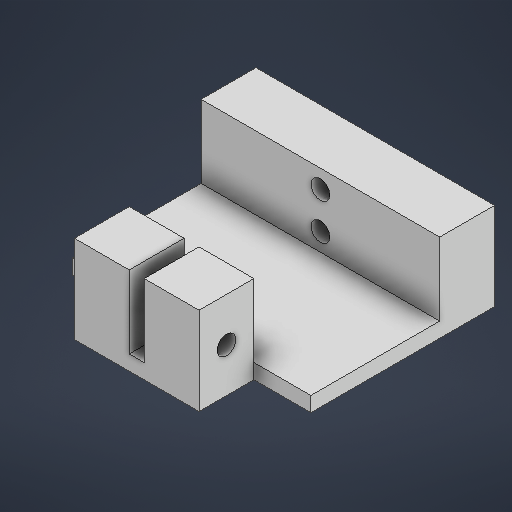
# Autodesk Inventor part: Slit holder
Saved by Autodesk Inventor 2027 (Build 310192060, 192F)
## iProperties
Created: 2026-07-27
Part Number: Slit holder
Material: Generic
Document SubType Name: Modeling
Designer: blaze
Density: 1 g/cm^3
Appearance: Default
Author: blaze
Autodesk Inventor part; units mm, degrees
ref_plane "YZ Plane" through (0, 0, 0) normal (1, 0, 0) x (0, 1, 0)
ref_plane "XZ Plane" through (0, 0, 0) normal (0, 1, 0) x (-1, 0, 0)
ref_plane "XY Plane" through (0, 0, 0) normal (0, 0, 1) x (1, 0, 0)
sketch "Sketch1" plane through (0, 0, 0) normal (0, 0, 1) x (1, 0, 0)
  line L0 (0, 0) -> (50.8, 0)
  line L1 (50.8, 0) -> (50.8, 18.669)
  line L2 (50.8, 18.669) -> (0, 18.669)
  line L3 (0, 18.669) -> (0, 0)
  dimension "d0" = 50.8
  dimension "d1" = 18.669
  constraints: 8 end point, 2 parallel, 1 horizontal, 1 perpendicular
  measures "d0" distance of L2.end L1.end
  measures "d1" distance of L1.end L0.end
extrude "Extrusion1" add sketch "Sketch1" against normal blind 50.8
sketch "Sketch2" plane through (0, 0, 0) normal (0, 0, 1) x (1, 0, 0)
  line L0 (50.8, 0) -> (0, 0) projected
  line L1 (25.4, 0) -> (25.4, 3.175)
  line L2 (25.4, 3.175) -> (26.9875, 3.175)
  line L3 (25.4, 3.175) -> (23.8125, 3.175)
  line L4 (23.8125, 3.175) -> (23.8125, 18.669)
  line L5 (0, 18.669) -> (50.8, 18.669) projected
  line L6 (26.9875, 3.175) -> (26.9875, 18.669)
  line L7 (23.8125, 18.669) -> (12.1285, 18.669)
  line L8 (12.1285, 18.669) -> (12.1285, 0)
  line L9 (12.1285, 0) -> (25.4, 0)
  line L10 (26.9875, 18.669) -> (38.6715, 18.669)
  line L11 (38.6715, 18.669) -> (38.6715, 0)
  line L12 (38.6715, 0) -> (25.4, 0)
  line L13 (0, 0) -> (0, 18.669) projected
  line L14 (0, 18.669) -> (0, 0)
  line L15 (50.8, 18.669) -> (50.8, 0) projected
  line L16 (50.8, 18.669) -> (50.8, 0)
  dimension "d4" = 3.175
  dimension "d5" = 1.5875
  dimension "d6" = 1.5875
  dimension "d15" = 11.684
  dimension "d16" = 11.684
  constraints: 26 end point, 6 point on line, 5 perpendicular, 3 vertical, 2 collinear, 1 horizontal, 1 midpoint
  measures "d4" distance of L1.start L1.end
  measures "d5" distance of L1.end L2.end
  measures "d6" distance of L1.end L3.end
  measures "d15" distance of L4.end L7.end
  measures "d16" distance of L6.end L10.end
sketch "Sketch3" plane through (0, 0, 0) normal (-1, 0, 0) x (0, 0, 1)
  line L0 (0, 0) -> (-50.8, 0) projected
  line L1 (0, 0) -> (0, 3.175)
  line L2 (0, 0) -> (0, 18.669) projected
  line L3 (0, 3.175) -> (-11.684, 3.175)
  line L4 (-50.8, 18.669) -> (-50.8, 0) projected
  line L5 (-50.8, 0) -> (-50.8, 3.175)
  line L6 (-50.8, 3.175) -> (-39.116, 3.175)
  line L7 (0, 18.669) -> (-50.8, 18.669) projected
  line L8 (-39.116, 3.175) -> (-11.684, 3.175)
  line L9 (-11.684, 3.175) -> (-11.684, 18.669)
  line L10 (-11.684, 18.669) -> (-39.116, 18.669)
  line L11 (-39.116, 18.669) -> (-39.116, 3.175)
  dimension "d7" = 3.175
  dimension "d8" = 11.684
  dimension "d9" = 3.175
  dimension "d10" = 11.684
  constraints: 16 end point, 3 perpendicular, 3 point on line, 2 parallel, 1 horizontal
  measures "d7" distance of L0.start L1.end
  measures "d8" distance of L1.end L3.end
  measures "d9" distance of L0.end L5.end
  measures "d10" distance of L5.end L6.end
extrude "Extrusion2" cut sketch "Sketch3" against normal blind 50.8 contours L8 L11 L7 L9
extrude "Extrusion3" cut sketch "Sketch2" against normal up to surface (11.684 mm away) contours L0 L11 L5 L15 | L0 L13 L5 L8
extrude "Extrusion4" cut sketch "Sketch2" against normal up to surface (11.684 mm away) contours L3 L4 L5 L6 L2
sketch "Sketch5" plane through (38.6715, 0, 0) normal (1, 0, 0) x (0, 0, -1)
  line L0 (0, 18.669) -> (11.684, 18.669) projected
  circle A0 centre (5.842, 9.3345) radius 2
  point P0 (0, 0)
  dimension "d21" = 4
  constraints: 1 centre point
  measures "d21" diameter of A0
extrude "Extrusion5" cut sketch "Sketch5" against normal up to surface (11.684 mm away)
sketch "Sketch6" plane through (0, 0, -50.8) normal (0, 0, -1) x (-1, 0, 0)
  line L0 (-50.8, 18.669) -> (-50.8, 0) projected
  line L1 (0, 18.669) -> (-50.8, 18.669) projected
  line L2 (-12.1285, 0) -> (-38.6715, 0) projected
  circle A0 centre (-25.4, 6.985) radius 2
  circle A1 centre (-25.4, 14.732) radius 2
  point P0 (0, 0)
  dimension "d25" = 4
  dimension "d27" = 4
  constraints: 2 centre point
  measures "d25" diameter of A0
  measures "d27" diameter of A1
extrude "Extrusion6" cut sketch "Sketch6" against normal up to surface (11.684 mm away)
body "Solid1"
